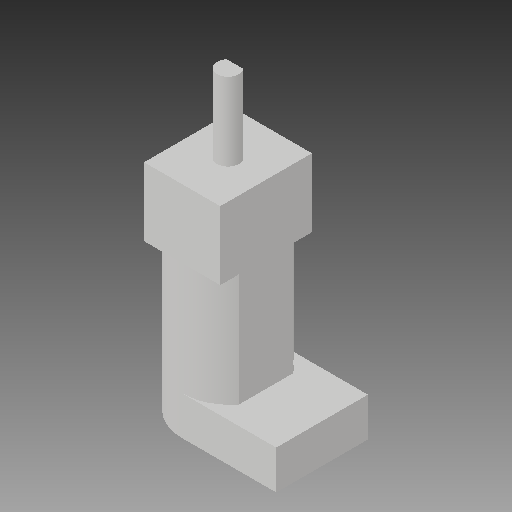
# Autodesk Inventor part: moteur
Saved by Autodesk Inventor 2019 (Build 230136000, 136)
## iProperties
Created: 2018-07-19
Part Number: moteur
Material: Générique
Document SubType Name: Modeling
Designer: julien.allali
Density: 1 g/cm^3
Appearance: Par défaut
Author: julien.allali
Autodesk Inventor part; units mm, degrees
ref_plane "YZ Plane" through (0, 0, 0) normal (1, 0, 0) x (0, 1, 0)
ref_plane "XZ Plane" through (0, 0, 0) normal (0, 1, 0) x (-1, 0, 0)
ref_plane "XY Plane" through (0, 0, 0) normal (0, 0, 1) x (1, 0, 0)
sketch "Sketch1" plane through (0, 0, 0) normal (0, 1, 0) x (-1, 0, 0)
  line L0 (0, 0) -> (9.8, 0)
  line L1 (9.8, 0) -> (9.8, -11.8)
  line L2 (9.8, -11.8) -> (0, -11.8)
  line L3 (0, -11.8) -> (0, 0)
  dimension "d0" = 11.8
  dimension "d1" = 9.8
  constraints: 8 end point, 2 parallel, 1 horizontal, 1 perpendicular
  measures "d0" distance of L0.end L1.end
  measures "d1" distance of L1.end L2.end
extrude "Extrusion1" add sketch "Sketch1" along normal blind 8.8
sketch "Sketch2" plane through (0, 8.8, 0) normal (0, 1, 0) x (1, 0, 0)
  circle A0 centre (-4.9, 5.9) radius 1.4
  line L0 (-9.8, 0) -> (0, 0) construction
  line L1 (0, 0) -> (0, 11.8) construction
  line L2 (0, 11.8) -> (-9.8, 11.8) construction
  line L3 (-9.8, 11.8) -> (-9.8, 0) construction
  line L4 (0, 11.8) -> (-9.8, 11.8) construction
  line L5 (-4.9, 11.8) -> (-4.9, 0) construction
  line L6 (-9.8, 0) -> (0, 0) construction
  line L7 (-9.8, 11.8) -> (-9.8, 0) construction
  line L8 (-9.8, 5.9) -> (0, 5.9) construction
  line L9 (0, 0) -> (0, 11.8) construction
  line L10 (-5.9724, 6.8) -> (-3.8276, 6.8)
  point P0 (-4.9, 5.9)
  dimension "d4" = 2.8
  dimension "d5" = 0.9
  constraints: 6 end point, 5 midpoint, 2 point on circle, 1 centre point, 1 coincident, 1 perpendicular
  measures "d4" diameter of A0
  measures "d5" distance between parallel lines of L8 L10
extrude "Extrusion2" add sketch "Sketch2" along normal blind 10 contours A0 L10 picked at (-5.0611, 5.8774)
sketch "Sketch3" plane through (0, 0, 0) normal (0, -1, 0) x (1, 0, 0)
  line L0 (0, 0) -> (0, -11.8) projected
  line L1 (0, -2.4) -> (0, -9.4)
  line L2 (-9.8, -11.8) -> (-9.8, 0) projected
  line L3 (-9.8, -2.4) -> (-9.8, -9.4)
  arc A0 (0, -2.4) -> (-9.8, -2.4) centre (-4.9, -6.2021) ccw
  arc A1 (-9.8, -9.4) -> (0, -9.4) centre (-4.9, -5.5979) ccw
  line L4 (-9.8, 0) -> (0, 0) projected
  line L5 (0, -11.8) -> (-9.8, -11.8) projected
  point P0 (0, -5.9)
  point P1 (-9.8, -5.9)
  point P2 (-4.9, 0)
  point P3 (-4.9, -11.8)
  dimension "d8" = 7
  dimension "d9" = 7
  constraints: 6 midpoint, 6 point on circle, 4 end point, 4 point on line, 2 centre point
  measures "d8" distance of L3.start L3.end
  measures "d9" distance of L1.start L1.end
extrude "Extrusion3" add sketch "Sketch3" along normal blind 14.5 contours L0 A1 L2 A0
sketch "Sketch4" plane through (0, -14.5, 0) normal (0, -1, 0) x (1, 0, 0)
  arc A0 (0, -2.4) -> (-9.8, -2.4) centre (-4.9, -6.2021) ccw projected
  line L0 (-9.8, -2.4) -> (-9.8, -9.4) projected
  arc A1 (-9.8, -9.4) -> (0, -9.4) centre (-4.9, -5.5979) ccw projected
  line L1 (0, -9.4) -> (0, -2.4) projected
  line L2 (-9.8, 0) -> (0, 0) projected
  line L3 (-4.9, 0) -> (7.2, 0)
  line L4 (7.2, 0) -> (7.2, -11.8)
  line L5 (7.2, -11.8) -> (-4.9, -11.8)
  line L6 (-4.9, -11.8) -> (-4.9, 0)
  dimension "d12" = 17
  constraints: 8 end point, 2 parallel, 1 horizontal, 1 midpoint, 1 perpendicular, 1 point on circle
  measures "d12" distance between parallel lines of L4 L0
extrude "Extrusion4" add sketch "Sketch4" along normal blind 5
body "Solid1"
